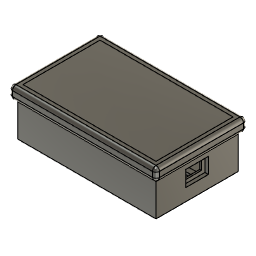
RFID-Case (Autodesk Fusion 360 design; units mm, degrees)
Autodesk Fusion 360 part; units mm, degrees
note: some values were not read from the file. Set by a fixed rule: which face or edge a step refers to.
sketch "Skizze1" plane through (0, 0, 0) normal (0, 0, 1) x (1, 0, 0)
  line L0 (0, 0) -> (76, 0)
  line L1 (76, 0) -> (76, 44)
  line L2 (76, 44) -> (0, 44)
  line L3 (0, 44) -> (0, 0)
  dimension "d1" = 76
  dimension "d2" = 44
  constraint horizontal L0
  constraint vertical L1
  constraint horizontal L2
  constraint vertical L3
  constraint coincident L0.start L3.end
  measures "d1" distance of L0.start L0.end
  measures "d2" distance of L0.start L2.end
extrude "Extrusion1" add sketch "Skizze1" along normal blind 27 makes body 1
shell "Schale1" thickness 1.5 removed faces 0 bodies 1
ref_plane "Arbeitsebene1" through (38, 22, 18) normal (0, 0, 1) x (1, 0, 0)
split "Teilen1" by plane through (38, 22, 18) normal (0, 0, 1) bodies 1 makes body 2 at (25.3333, 29.3333, 27)
copy_body "Körper->Berechn1" bodies 1 removing the originals makes body 3 in component "Box"
copy_body "Körper->Berechn2" bodies 2 removing the originals makes body 4 in component "Deckel"
sketch "Skizze2" plane through (0, 0, 25.5) normal (0, 0, -1) x (1, 0, 0)
  line L0 (1.5, -1.5) -> (1.5, -42.5)
  line L1 (1.5, -42.5) -> (74.5, -42.5)
  line L2 (74.5, -42.5) -> (74.5, -1.5)
  line L3 (74.5, -1.5) -> (1.5, -1.5)
  line L4 (67.7, -9.1) -> (30.7, -9.1) construction
  line L5 (30.7, -9.1) -> (30.7, -34.9) construction
  line L6 (30.7, -34.9) -> (67.7, -34.9) construction
  line L7 (67.7, -34.9) -> (67.7, -9.1) construction
  circle A0 centre (67.7, -9.1) radius 1.25
  circle A1 centre (67.7, -34.9) radius 1.25
  circle A2 centre (67.7, -9.1) radius 2.5
  circle A3 centre (67.7, -34.9) radius 2.5
  circle A4 centre (30.7, -5.1) radius 2.5
  circle A5 centre (30.7, -38.9) radius 2.5
  circle A6 centre (30.7, -5.1) radius 1.25
  circle A7 centre (30.7, -38.9) radius 1.25
  dimension "d7" = 6.8
  dimension "d8" = 7.6
  dimension "d9" = 25.8
  dimension "d10" = 2.5
  dimension "d11" = 5
  dimension "d12" = 37
  dimension "d13" = 4
  dimension "d14" = 4
  dimension "d15" = 5
  constraint horizontal L4
  constraint vertical L5
  constraint horizontal L6
  constraint vertical L7
  constraint coincident L4.start L7.end
  constraint coincident L6.end L7.start
  constraint equal A0 A1
  constraint concentric A0 A2
  constraint equal A2 A3
  constraint equal A4 A5
  constraint vertical L4.end A4.centre
  constraint vertical L5.end A5.centre
  constraint concentric A4 A6
  constraint concentric A5 A7
  constraint equal A0 A6
  constraint equal A0 A7
  measures "d7" distance of L2 L7
  measures "d8" distance of L3 L4.start
  measures "d9" distance of L4.start L6.end
  measures "d10" diameter of A0
  measures "d11" diameter of A2
  measures "d12" distance of L4.start L4.end
  measures "d13" distance of L4.end A4.centre
  measures "d14" distance of L5.end A5.centre
  measures "d15" diameter of A4
extrude "Extrusion1'" add sketch "Skizze2" along normal blind 5 contours A2 | A3 | A4 | A5 bodies 4 in component "Deckel"
extrude "Extrusion2" add sketch "Skizze2" along normal blind 2 contours A0 | A1 | A6 | A7 bodies 4 in component "Deckel"
sketch "Skizze3" plane through (76, 0, 0) normal (1, 0, 0) x (0, 1, 0)
  line L0 (44, 18) -> (0, 18)
  line L1 (0, 18) -> (0, 0)
  line L2 (0, 0) -> (44, 0)
  line L3 (44, 0) -> (44, 18)
  line L4 (17.5, 14) -> (26.5, 14)
  line L5 (26.5, 14) -> (26.5, 9)
  line L6 (26.5, 9) -> (17.5, 9)
  line L7 (17.5, 9) -> (17.5, 14)
  line L8 (22, 0) -> (22, 18) construction
  dimension "d20" = 9
  dimension "d21" = 5
  dimension "d22" = 4
  constraint horizontal L4
  constraint vertical L5
  constraint horizontal L6
  constraint vertical L7
  constraint midpoint L2 L8.start
  constraint midpoint L0 L8.end
  constraint symmetric L5 L7 L8
  measures "d20" distance of L5.end L6.end
  measures "d21" distance of L4.end L5.end
  measures "d22" distance of L0 L4.start
extrude "Extrusion1''" cut sketch "Skizze3" against normal up to surface (1.5 mm away) contours L4 L5 L6 L7 bodies 3 in component "Box"
sketch "Skizze4" plane through (38, 22, 18) normal (0, 0, 1) x (1, 0, 0)
  line L0 (38, -22) -> (38, 22)
  line L1 (38, 22) -> (-38, 22)
  line L2 (-38, -22) -> (38, -22)
  line L3 (-38, 22) -> (-38, -22)
  line L4 (39.5, -23.5) -> (39.5, 23.5)
  line L5 (39.5, 23.5) -> (-39.5, 23.5)
  line L6 (-39.5, 23.5) -> (-39.5, -23.5)
  line L7 (-39.5, -23.5) -> (39.5, -23.5)
  dimension "d27" = 1.5
extrude "Extrusion2'" add sketch "Skizze4" along normal blind 2 and the other way up to surface (18 mm away) bodies 3 in component "Box"
sketch "Skizze5" plane through (77.5, 0, 0) normal (1, 0, 0) x (0, 1, 0)
  line L0 (45.5, 0) -> (45.5, 20)
  line L1 (45.5, 20) -> (-1.5, 20)
  line L2 (-1.5, 20) -> (-1.5, 0)
  line L3 (-1.5, 0) -> (45.5, 0)
  line L4 (17.5, 14) -> (17.5, 9)
  line L5 (17.5, 9) -> (26.5, 9)
  line L6 (26.5, 9) -> (26.5, 14)
  line L7 (26.5, 14) -> (17.5, 14)
  line L8 (1.5, 18) -> (42.5, 18)
  line L9 (42.5, 18) -> (42.5, 1.5)
  line L10 (42.5, 1.5) -> (1.5, 1.5)
  line L11 (1.5, 1.5) -> (1.5, 18)
  line L12 (28.5, 16) -> (15.5, 16)
  line L13 (15.5, 16) -> (15.5, 7)
  line L14 (15.5, 7) -> (28.5, 7)
  line L15 (28.5, 7) -> (28.5, 16)
  dimension "d32" = 2
extrude "Extrusion3" cut sketch "Skizze5" against normal blind 2 contours L4 L5 L6 L7 | L12 L13 L14 L15 bodies 3 in component "Box"
sketch "Skizze6" plane through (0, 0, 1.5) normal (0, 0, 1) x (-1, 0, 0)
  line L0 (-1.5, -42.5) -> (-1.5, -1.5)
  line L1 (-1.5, -1.5) -> (-74.5, -1.5)
  line L2 (-74.5, -1.5) -> (-74.5, -42.5)
  line L3 (-74.5, -42.5) -> (-1.5, -42.5)
  line L4 (-74.5, -13.5) -> (-1.5, -13.5)
  line L5 (-1.5, -13.5) -> (-1.5, -16.5)
  line L6 (-1.5, -16.5) -> (-74.5, -16.5)
  line L7 (-74.5, -16.5) -> (-74.5, -13.5)
  line L8 (-74.5, -27.5) -> (-1.5, -27.5)
  line L9 (-1.5, -27.5) -> (-1.5, -30.5)
  line L10 (-1.5, -30.5) -> (-74.5, -30.5)
  line L11 (-74.5, -30.5) -> (-74.5, -27.5)
  dimension "d35" = 3
  dimension "d36" = 3
  dimension "d37" = 12
  dimension "d38" = 12
  constraint horizontal L4
  constraint vertical L5
  constraint horizontal L6
  constraint vertical L7
  constraint coincident L0 L5.end
  constraint coincident L2 L4.start
  constraint horizontal L8
  constraint vertical L9
  constraint horizontal L10
  constraint vertical L11
  constraint coincident L0 L9.end
  constraint coincident L2 L8.start
  measures "d35" distance of L4 L6
  measures "d36" distance of L8 L10
  measures "d37" distance of L2.end L10.end
  measures "d38" distance of L1.end L4.start
extrude "Extrusion4" add sketch "Skizze6" along normal blind 1.4 contours L0 L2 L8 L9 L10 L11 | L0 L2 L4 L5 L6 L7 bodies 3 in component "Box"
fillet "Abrundung1" radius 1.5 4 edges at (-1.5, 22, 20) (38, -1.5, 20) (38, 45.5, 20) (77.5, 22, 20) on bodies 3 in component "Box"
sketch "Skizze1 (2)" plane through (0, 0, 27) normal (0, 0, 1) x (-1, 0, 0) in component "Blende"
  line L0 (0, -44) -> (0, 0)
  line L1 (0, 0) -> (-76, 0)
  line L2 (-76, 0) -> (-76, -44)
  line L3 (-76, -44) -> (0, -44)
  line L4 (0, -44) -> (-76, -44)
  line L5 (-76, -44) -> (-76, 0)
  line L6 (-76, 0) -> (0, 0)
  line L7 (0, 0) -> (0, -44)
  line L8 (-80, 4) -> (4, 4)
  line L9 (4, 4) -> (4, -48)
  line L10 (4, -48) -> (-80, -48)
  line L11 (-80, -48) -> (-80, 4)
  dimension "d43" = -4
  constraint horizontal L4
  constraint vertical L5
  constraint horizontal L6
  constraint vertical L7
  constraint coincident L1.end L2.start
  constraint coincident L0.start L3.end
extrude "Extrusion1'''" add sketch "Skizze1 (2)" against normal blind 7 separate body makes body 5 in component "Blende"
fillet "Abrundung1'" radius 2 12 edges at (38, 48, 20) (-4, 22, 20) (38, -4, 20) (80, 22, 20) (80, -4, 23.5) (-4, -4, 23.5) (80, 48, 23.5) (-4, 48, 23.5) (-4, 22, 27) (38, 48, 27) (38, -4, 27) (80, 22, 27) on bodies 5 in component "Blende"
component "Box" placed x (1, 0, 0) y (0, 1, 0) z (0, 0, 1) at (0, 0, 0)
component "Deckel" placed x (1, 0, 0) y (0, 1, 0) z (0, 0, 1) at (0, 0, 0)
component "Blende" placed x (1, 0, 0) y (0, 1, 0) z (0, 0, 1) at (0, 0, 0)
equation "d8 = ( ( 41 - 25.8 ) / 2 ) * 1 mm"
equation "d14 = d13"
equation "d36 = d35"
